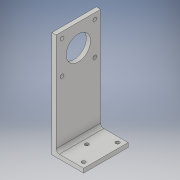
# Autodesk Inventor part: Suporte Esquerdo
Saved by Autodesk Inventor 2017 (Build 210142000, 142)
## iProperties
Created: 2016-07-16
Part Number: Suporte Esquerdo
Material: Generic
Document SubType Name: Modeling
Designer: mateu
Density: 1 g/cm^3
Appearance: Default
Author: mateu
Autodesk Inventor part; units mm, degrees
ref_plane "YZ Plane" through (0, 0, 0) normal (1, 0, 0) x (0, 1, 0)
ref_plane "XZ Plane" through (0, 0, 0) normal (0, 1, 0) x (-1, 0, 0)
ref_plane "XY Plane" through (0, 0, 0) normal (0, 0, 1) x (1, 0, 0)
sketch "Sketch1" plane through (0, 0, 0) normal (0, 0, 1) x (1, 0, 0)
  line L0 (0, 0) -> (0, -100)
  line L1 (0, -100) -> (30, -100)
  line L2 (30, -100) -> (30, -96)
  line L3 (30, -96) -> (4, -96)
  line L4 (4, -96) -> (4, 0)
  line L5 (4, 0) -> (0, 0)
  dimension "d0" = 100
  dimension "d1" = 30
  dimension "d2" = 4
  dimension "d3" = 26
  constraints: 12 end point, 5 perpendicular, 1 vertical
  measures "d0" distance of L0.start L0.end
  measures "d1" distance of L0.end L1.end
  measures "d2" distance of L1.end L2.end
  measures "d3" distance of L2.end L3.end
extrude "Extrusion1" add sketch "Sketch1" along normal blind 42
sketch "Sketch2" plane through (4, -96, 0) normal (1, 0, 0) x (0, 0, -1)
  line L0 (-42, 96) -> (-42, -4) projected
  line L1 (0, 96) -> (0, -4) projected
  line L2 (-42, 96) -> (0, 96)
  line L3 (0, 96) -> (0, 0)
  line L4 (0, 0) -> (-42, 0)
  line L5 (-42, 0) -> (-42, 96)
  circle A0 centre (-36.5, 90.5) radius 1.75
  circle A1 centre (-5.5, 90.5) radius 1.75
  circle A2 centre (-36.5, 59.5) radius 1.75
  circle A3 centre (-5.5, 59.5) radius 1.75
  circle A4 centre (-21, 75) radius 11.5
  dimension "d6" = 96
  dimension "d7" = 3.5
  dimension "d8" = 5.5
  dimension "d9" = 5.5
  dimension "d10" = 3.5
  dimension "d11" = 5.5
  dimension "d12" = 5.5
  dimension "d14" = 3.5
  dimension "d15" = 3.5
  dimension "d16" = 31
  dimension "d17" = 31
  dimension "d18" = 5.5
  dimension "d19" = 5.5
  dimension "d20" = 23
  dimension "d21" = 21
  dimension "d22" = 15.5
  constraints: 8 end point, 5 centre point, 2 parallel, 1 horizontal, 1 perpendicular, 1 point on line
  measures "d6" distance of L2.end L3.end
  measures "d7" diameter of A0
  measures "d8" distance from line of L0 A0.centre
  measures "d9" distance from line of L2 A0.centre
  measures "d10" diameter of A1
  measures "d11" distance from line of L1 A1.centre
  measures "d12" distance from line of L2 A1.centre
  measures "d14" diameter of A2
  measures "d15" diameter of A3
  measures "d16" distance of A2.centre A0.centre
  measures "d17" distance of A3.centre A1.centre
  measures "d18" distance from line of L0 A2.centre
  measures "d19" distance from line of L1 A3.centre
  measures "d20" diameter of A4
  measures "d21" distance from line of L1 A4.centre
  measures "d22" horizontal distance of A1.centre A4.centre
extrude "Extrusion2" cut sketch "Sketch2" against normal blind 4 contours A0 | A1 | A2 | A3 | A4
sketch "Sketch3" plane through (4, -96, 0) normal (0, 1, 0) x (1, 0, 0)
  line L0 (-4, 0) -> (-4, -42) projected
  line L1 (26, 0) -> (26, -42) projected
  line L2 (-4, 0) -> (26, 0)
  line L3 (26, 0) -> (26, -42)
  line L4 (26, -42) -> (-4, -42)
  line L5 (-4, -42) -> (-4, 0)
  circle A0 centre (21, -5) radius 1.75
  circle A1 centre (21, -37) radius 1.75
  circle A2 centre (8, -21) radius 1.75
  dimension "d25" = 3.5
  dimension "d26" = 3.5
  dimension "d27" = 3.5
  dimension "d28" = 5
  dimension "d29" = 5
  dimension "d30" = 5
  dimension "d31" = 5
  dimension "d32" = 12
  dimension "d33" = 21
  constraints: 8 end point, 3 centre point, 2 parallel, 1 horizontal, 1 perpendicular
  measures "d25" diameter of A0
  measures "d26" diameter of A1
  measures "d27" diameter of A2
  measures "d28" distance from line of L1 A0.centre
  measures "d29" distance from line of L2 A0.centre
  measures "d30" distance from line of L4 A1.centre
  measures "d31" distance from line of L1 A1.centre
  measures "d32" distance from line of L0 A2.centre
  measures "d33" distance from line of L2 A2.centre
extrude "Extrusion3" cut sketch "Sketch3" against normal blind 4 contours A0 | A1 | A2
fillet "Fillet1" radius 3 1 edges at (4, -96, 21)
body "Solid1"
